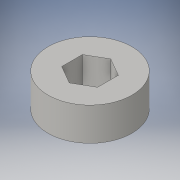
# Autodesk Inventor part: 3-8th inch hex shaft collar
Saved by Autodesk Inventor 2016 (Build 200138000, 138)
## iProperties
Created: 2016-02-06
Part Number: 3-8th inch hex shaft collar
Material: Generic
Document SubType Name: Modeling
Designer: gus
Density: 1 g/cm^3
Appearance: Default
Author: gus
Autodesk Inventor part; units mm, degrees
ref_plane "YZ Plane" through (0, 0, 0) normal (1, 0, 0) x (0, 1, 0)
ref_plane "XZ Plane" through (0, 0, 0) normal (0, 1, 0) x (-1, 0, 0)
ref_plane "XY Plane" through (0, 0, 0) normal (0, 0, 1) x (1, 0, 0)
sketch "Sketch1" plane through (0, 0, 0) normal (0, 1, 0) x (-1, 0, 0)
  circle A0 centre (0, 0) radius 11.1125
  line L0 (0, -5.4993) -> (-4.7625, -2.7496)
  line L1 (-4.7625, -2.7496) -> (-4.7625, 2.7496)
  line L2 (-4.7625, 2.7496) -> (0, 5.4993)
  line L3 (0, 5.4993) -> (4.7625, 2.7496)
  line L4 (4.7625, 2.7496) -> (4.7625, -2.7496)
  line L5 (4.7625, -2.7496) -> (0, -5.4993)
  dimension "d0" = 22.225
  dimension "d1" = 9.525
  constraints: 12 end point, 2 coincident, 1 centre point, 1 vertical, 13 other
  measures "d0" diameter of A0
  measures "d1" distance between parallel lines of L1 L4
extrude "Extrusion1" add sketch "Sketch1" along normal blind 8.763
body "Solid1"
